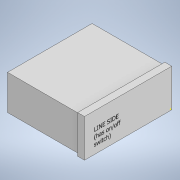
# Autodesk Inventor part: Power_entry_AK_or_AR_2
Saved by Autodesk Inventor 2020 (Build 240168000, 168)
## iProperties
Created: 2020-01-13
Part Number: Power_entry_AK_or_AR_2
Material: Generic
Document SubType Name: Modeling
Designer: ColinP
Density: 1 g/cm^3
Appearance: Default
Author: ColinP
Autodesk Inventor part; units mm, degrees
ref_plane "YZ Plane" through (0, 0, 0) normal (1, 0, 0) x (0, 1, 0)
ref_plane "XZ Plane" through (0, 0, 0) normal (0, 1, 0) x (-1, 0, 0)
ref_plane "XY Plane" through (0, 0, 0) normal (0, 0, 1) x (1, 0, 0)
sketch "Sketch1" plane through (0, 0, 0) normal (0, 1, 0) x (-1, 0, 0)
  line L0 (0, 0) -> (0, 65.278)
  line L1 (0, 65.278) -> (55.118, 65.278)
  line L2 (55.118, 65.278) -> (55.118, 0)
  line L3 (55.118, 0) -> (0, 0)
  dimension "d0" = 65.278
  dimension "d1" = 55.118
  constraints: 8 end point, 2 perpendicular, 2 vertical
  measures "d0" distance of L0.start L0.end
  measures "d1" distance of L0.end L1.end
extrude "Extrusion1" add sketch "Sketch1" along normal blind 26.8986
sketch "Sketch2" plane through (0, 0, 65.278) normal (1, 0, 0) x (0, 0, -1)
  line L0 (65.278, 26.8986) -> (0, 26.8986) projected
  line L1 (65.278, 0) -> (0, 0) projected
  line L2 (0, 0) -> (0, -1.1557)
  line L3 (0, -1.1557) -> (-1.016, -1.1557)
  line L4 (-1.016, -1.1557) -> (-1.016, 28.0543)
  line L5 (-1.016, 28.0543) -> (66.294, 28.0543)
  line L6 (66.294, 28.0543) -> (66.294, -1.1557)
  line L7 (66.294, -1.1557) -> (0, -1.1557)
  dimension "d7" = 1.1557
  dimension "d8" = 1.016
  dimension "d9" = 29.21
  dimension "d10" = 67.31
  constraints: 12 end point, 4 perpendicular, 1 horizontal, 1 point on line, 1 vertical
  measures "d7" distance of L1.end L2.end
  measures "d8" distance of L2.end L3.end
  measures "d9" distance of L3.end L4.end
  measures "d10" distance of L4.end L5.end
extrude "Extrusion2" add sketch "Sketch2" along normal blind 5.334
sketch "Sketch3" plane through (5.334, 0, 65.278) normal (1, 0, 0) x (0, 0, -1)
  line L0 (6.2473, 17.0204) -> (32.1207, 17.0204) construction
  line L1 (32.1207, 17.0204) -> (32.1207, 13.8637) construction
  line L2 (32.1207, 13.8637) -> (6.2473, 13.8637) construction
  line L3 (6.2473, 13.8637) -> (6.2473, 17.0204) construction
  point P0 (65.278, 0)
  constraints: 2 other
sketch "Sketch4" plane through (-55.118, 0, 0) normal (-1, 0, 0) x (0, 0, 1)
  line L0 (-2.6118, 20.4476) -> (65.0145, 20.4476) construction
  line L1 (65.0145, 20.4476) -> (65.0145, -8.8115) construction
  line L2 (65.0145, -8.8115) -> (-2.6118, -8.8115) construction
  line L3 (-2.6118, -8.8115) -> (-2.6118, 20.4476) construction
  point P0 (0, 0)
  constraints: 2 other
body "Solid1"
